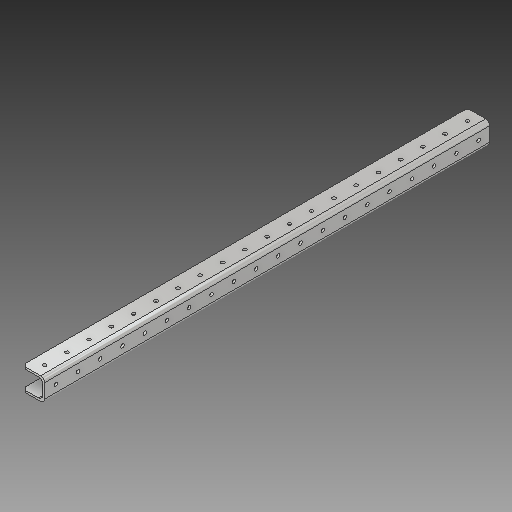
# Autodesk Inventor part: channel-1x1x1-0001
Saved by Autodesk Inventor 2018 (Build 220112000, 112)
## iProperties
Created: 2016-07-01
Part Number: channel-1x1x1-0001
Material: Aluminum 5052-H36
Document SubType Name: Modeling
Designer: rickab1
Density: 2.68277 g/cm^3
Appearance: Aluminum - Polished
Author: rickab1
Autodesk Inventor part; units mm, degrees
ref_plane "YZ Plane" through (0, 0, 0) normal (1, 0, 0) x (0, 1, 0)
ref_plane "XZ Plane" through (0, 0, 0) normal (0, 1, 0) x (-1, 0, 0)
ref_plane "XY Plane" through (0, 0, 0) normal (0, 0, 1) x (1, 0, 0)
sketch "Sketch1" plane through (0, 0, 0) normal (0, 0, 1) x (1, 0, 0)
  line L0 (-12.7, -12.7) -> (12.7, -12.7)
  line L1 (12.7, -12.7) -> (12.7, 12.7)
  line L2 (12.7, 12.7) -> (-12.7, 12.7)
  line L3 (-12.7, -12.7) -> (12.7, 12.7) construction
  line L4 (12.7, -12.7) -> (-12.7, 12.7) construction
  line L5 (-12.7, 10.414) -> (10.414, 10.414)
  line L6 (10.414, 10.414) -> (10.414, -10.414)
  line L7 (10.414, -10.414) -> (-12.7, -10.414)
  line L8 (-12.7, 10.414) -> (-12.7, 12.7)
  line L9 (-12.7, -10.414) -> (-12.7, -12.7)
  point P0 (0, 0)
  dimension "l1" = 25.4
  dimension "l2" = 25.4
  dimension "wt" = 2.286
  constraints: 20 end point, 3 vertical alignment, 2 midpoint, 2 parallel, 2 perpendicular, 2 vertical, 1 horizontal, 2 other
  measures "l1" distance of L1.end L2.end
  measures "l2" distance of L0.end L1.end
  measures "wt" distance between parallel lines of L0 L7
extrude "Extrusion1" add sketch "Sketch1" against normal blind 508
sketch "Sketch2" plane through (-12.7, 12.7, 0) normal (0, 1, 0) x (1, 0, 0)
  line L0 (25.4, 0) -> (0, 0) projected
  line L1 (25.4, 0) -> (25.4, 508) projected
  line L2 (0, 508) -> (25.4, 508) projected
  line L3 (0, 0) -> (0, 508) projected
  point P0 (12.7, 0)
  point P1 (12.7, 12.7)
  dimension "d5" = 25.4
  dimension "d7" = 12.7
  dimension "d8" = 12.7
  measures "d5" distance of L0.start L0.end
  measures "d7" distance from line of L1 point (12.7, 12.7)
  measures "d8" distance from line of L0 point (12.7, 12.7)
hole "Hole1" at (0, 12.7, -12.7) direction (0, -1, 0) diameter 4.0894 end through all
sketch "Sketch3" plane through (12.7, -12.7, 0) normal (1, 0, 0) x (0, 0, -1)
  line L0 (0, 0) -> (0, 25.4) projected
  line L1 (0, 0) -> (508, 0) projected
  line L2 (508, 25.4) -> (508, 0) projected
  line L3 (0, 25.4) -> (508, 25.4) projected
  point P0 (0, 12.7)
  point P1 (12.7, 12.7)
  dimension "bot_dist" = 12.7
  dimension "d17" = 25.4
  dimension "d18" = 12.7
  measures "bot_dist" distance from line of L0 point (12.7, 12.7)
  measures "d17" distance of L0.start L0.end
  measures "d18" distance from line of L1 point (12.7, 12.7)
hole "Hole2" at (12.7, 0, -12.7) direction (-1, 0, 0) diameter 4.0894 end through all
sketch "Sketch4" plane through (12.7, -12.7, 0) normal (1, 0, 0) x (0, 0, -1)
  line L0 (0, 0) -> (0, 25.4) projected
  line L1 (0, 25.4) -> (508, 25.4) projected
  line L2 (0, 0) -> (508, 0) projected
  point P0 (0, 12.7)
  point P1 (12.7, 12.7)
  point P2 (12.7, 12.7)
  dimension "d26" = 12.7
  dimension "d27" = 12.7
  dimension "d28" = 12.7
  constraints: 1 coincident
  measures "d26" distance from line of L0 point (12.7, 12.7)
  measures "d27" distance from line of L1 point (12.7, 12.7)
  measures "d28" distance from line of L2 point (12.7, 12.7)
hole "Hole3" [suppressed]
pattern_linear "Rectangular Pattern1" count 21 spacing 25.4 along (0, 0, -1) of "Hole1"
pattern_linear "Rectangular Pattern2" count 21 spacing 25.4 along (0, 0, -1) of "Hole2"
pattern_linear "Rectangular Pattern3" [suppressed]
chamfer "Chamfer1" distance 3.175 angle 45 4 edges at (-12.7, 11.557, 0) (-12.7, -11.557, 0) (-12.7, 11.557, -508) (-12.7, -11.557, -508)
fillet "Fillet1" radius 4.572 4 edges at (12.7, 12.7, -254) (12.7, -12.7, -254) (10.414, -10.414, -254) (10.414, 10.414, -254)
equation "\"d7\" = 0.5 * d5"
equation "\"d18\" = 0.5 * d17"
body "Solid1"
